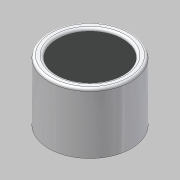
# Autodesk Inventor part: Parallax_Ping_Transducer
Saved by Autodesk Inventor 2012 (Build 160160000, 160)
## iProperties
Manager: Ed Sparks
Company: FirstCadLibrary
Shininess: 64.0
Length Units: 11269
Angle Units: 11279
Time Units: 11290
Mass Units: 11283
Length Display Precision: 3
Angle Display Precision: 2
Compacted: True
Part Number: Parallax_Ping_Transducer
Document SubType Name: Modeling
Created: 2007-12-18
Project: FIRST
Material: ABS Plastic
Catalog Web Link: www.firstcadlibrary.com
Designer: Ed Sparks
Engineer: Ed Sparks
Density: 1.06 g/cm^3
Mass: 2.57873 g
Surface Area: 10.3251 cm^2
Volume: 2.43276 cm^3
Density: 0.0
Volumn: 0.0
Area: 0.0
PropertySet Name: Model Information
Control State: 0
Master: False
Checked Out: False
Author: Ed Sparks
Keywords: FIRST
Autodesk Inventor part; units mm, degrees
ref_plane "YZ Plane" through (0, 0, 0) normal (1, 0, 0) x (0, 1, 0)
ref_plane "XZ Plane" through (0, 0, 0) normal (0, 1, 0) x (-1, 0, 0)
ref_plane "XY Plane" through (0, 0, 0) normal (0, 0, 1) x (1, 0, 0)
sketch "Sketch1" plane through (0, 0, 0) normal (0, 0, 1) x (1, 0, 0)
  circle A0 centre (0, 0) radius 8.15
  dimension "d0" = 16.3
  constraints: 1 centre point, 1 other
  measures "d0" diameter of A0
extrude "Extrusion1" add sketch "Sketch1" along normal blind 12
sketch "Sketch2" plane through (0, 0, 12) normal (0, 0, 1) x (1, 0, 0)
  circle A0 centre (0, 0) radius 8.15 projected
  constraints: 1 coincident
hole "Hole1" at (0, 0, 12) direction (0, 0, -1) diameter 13 depth 0.5
fillet "Fillet1" radius 0.5 2 edges at (-8.15, 0, 12) (0, 6.5, 12)
body "Solid1"
